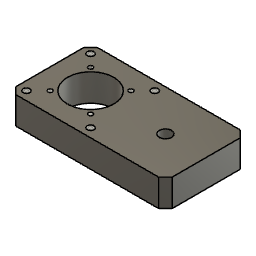
BC linear drive bottom bracket v13 (Autodesk Fusion 360 design; units mm, degrees)
Autodesk Fusion 360 part; units mm, degrees
note: some values were not read from the file. Set by a fixed rule: the direction of a hole.
sketch "Sketch1" plane through (0, 0, 0) normal (0, 1, 0) x (1, 0, 0)
  circle A0 centre (-55, 0) radius 17
  line L0 (-78.57, 23.57) -> (-31.43, 23.57) construction
  line L1 (-31.43, 23.57) -> (-31.43, -23.57) construction
  line L2 (-31.43, -23.57) -> (-78.57, -23.57) construction
  line L3 (-78.57, -23.57) -> (-78.57, 23.57) construction
  line L4 (-78.57, -23.57) -> (-31.43, 23.57) construction
  line L5 (-85, 30) -> (30, 30)
  line L6 (30, 30) -> (30, -30)
  line L7 (30, -30) -> (-85, -30)
  line L8 (-85, -30) -> (-85, 30)
  line L9 (0, 0) -> (-55, 0) construction
  circle A1 centre (-55, 0) radius 21 construction
  line L10 (-78.57, 23.57) -> (-31.43, -23.57) construction
  line L11 (-55, 23.57) -> (-55, -23.57) construction
  line L12 (-78.57, 0) -> (-31.43, 0) construction
  point P0 (-55, 21)
  point P1 (-69.8492, 14.8492)
  point P2 (-76, 0)
  point P3 (-69.8492, -14.8492)
  point P4 (-55, -21)
  point P5 (-40.1508, -14.8492)
  point P6 (-40.1508, 14.8492)
  point P7 (-34, 0)
  dimension "d2" = 34
  dimension "d3" = 55
  dimension "d4" = 47.14
  dimension "d5" = 30
  dimension "d6" = 30
  dimension "d7" = 60
  dimension "d20" = 42
  constraint horizontal L0
  constraint vertical L1
  constraint horizontal L2
  constraint vertical L3
  constraint equal L2 L3
  constraint midpoint A0.centre L4
  constraint horizontal L5
  constraint vertical L6
  constraint horizontal L7
  constraint vertical L8
  constraint coincident L9.start origin
  constraint coincident A0.centre L9.end
  constraint symmetric L5 L7 L9
  constraint midpoint L0 L11.start
  constraint midpoint L2 L11.end
  constraint midpoint L3 L12.start
  constraint midpoint L1 L12.end
  constraint coincident A1 P0
  constraint coincident L11 P0
  constraint coincident A1 P1
  constraint coincident L10 P1
  constraint coincident A1 P2
  constraint coincident L12 P2
  constraint coincident A1 P3
  constraint coincident L4 P3
  constraint coincident L11 P4
  constraint coincident A1 P4
  constraint coincident A1 P5
  constraint coincident L10 P5
  constraint coincident A1 P6
  constraint coincident L4 P6
  constraint coincident A1 P7
  constraint coincident L9 P7
  measures "d2" diameter of A0
  measures "d3" distance of L9.start A0.centre
  measures "d4" distance of L1.end L2.end
  measures "d5" distance of L9.start L6
  measures "d6" distance of A0.centre L8
  measures "d7" distance of L5.end L6.end
  measures "d20" diameter of A1
extrude "Extrude1" add sketch "Sketch1" along normal blind 20
hole "Hole1" at (0, 0, 0) direction (0, 1, 0) diameter 9 end through all
hole "Hole2" at (-31.43, 0, 23.57) at (-31.43, 0, -23.57) at (-78.57, 0, -23.57) at (-78.57, 0, 23.57) direction (0, 1, 0) diameter 5.029 end through all
thread "Thread3" "ISO Metric profile 5.5 M5.5x0.5 6H" thread offset 0 thread depth 10
hole "Hole3" at (-69.8492, 0, 14.8492) at (-69.8492, 0, -14.8492) at (-40.1508, 0, -14.8492) at (-40.1508, 0, 14.8492) direction (0, 1, 0) diameter 3.332 end through all
thread "Thread2" "ISO Metric profile 4.0 M4x0.7 6H" thread offset 0 thread depth 10
chamfer "Chamfer3" distance 5 angle 45 4 edges at (-85, 10, 30) (-85, 10, -30) (30, 10, 30) (30, 10, -30)
